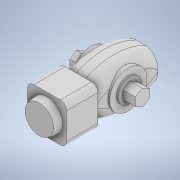
# Autodesk Inventor part: Weapon-Healing-Body
Saved by Autodesk Inventor 2020 (Build 240168000, 168)
## iProperties
Created: 2019-12-02
Part Number: Weapon-Healing-Body
Material: Generic
Document SubType Name: Modeling
Designer: vifly_01
Density: 1 g/cm^3
Appearance: Default
Author: vifly_01
Autodesk Inventor part; units mm, degrees
ref_plane "YZ Plane" through (0, 0, 0) normal (1, 0, 0) x (0, 1, 0)
ref_plane "XZ Plane" through (0, 0, 0) normal (0, 1, 0) x (-1, 0, 0)
ref_plane "XY Plane" through (0, 0, 0) normal (0, 0, 1) x (1, 0, 0)
sketch "Sketch1" plane through (0, 0, 0) normal (0, 0, 1) x (1, 0, 0)
  circle A0 centre (0, 0) radius 5
  dimension "d0" = 10
  constraints: 1 centre point, 1 coincident
  measures "d0" diameter of A0
extrude "Extrusion1" add sketch "Sketch1" along normal blind 2.5 draft -10
sketch "Sketch2" plane through (0, 0, 0) normal (0, 0, -1) x (-1, 0, 0)
  line L0 (-6.25, -6.25) -> (6.25, -6.25)
  line L1 (6.25, -6.25) -> (6.25, 6.25)
  line L2 (6.25, 6.25) -> (-6.25, 6.25)
  line L3 (-6.25, 6.25) -> (-6.25, -6.25)
  line L4 (-6.25, -6.25) -> (6.25, 6.25) construction
  line L5 (6.25, -6.25) -> (-6.25, 6.25) construction
  point P0 (0, 0)
  dimension "d3" = 12.5
  dimension "d4" = 12.5
  constraints: 12 end point, 2 midpoint, 2 parallel, 1 horizontal, 1 perpendicular
  measures "d3" distance of L2.end L1.end
  measures "d4" distance of L1.end L0.end
extrude "Extrusion2" add sketch "Sketch2" along normal blind 10
sketch "Sketch3" plane through (0, 0, 0) normal (1, 0, 0) x (0, 1, 0)
  line L0 (7.5, -10) -> (7.5, -30)
  line L1 (7.5, -30) -> (-7.5, -30)
  line L2 (-7.5, -30) -> (-7.5, -10)
  line L3 (-7.5, -10) -> (7.5, -10)
  point P0 (0, 0)
  dimension "d7" = 20
  dimension "d8" = 15
  constraints: 8 end point, 2 parallel, 1 perpendicular, 1 vertical
  measures "d7" distance of L0.start L0.end
  measures "d8" distance of L0.end L1.end
extrude "Extrusion3" add sketch "Sketch3" along normal mid plane 11
sketch "Sketch4" plane through (0, 0, 0) normal (1, 0, 0) x (0, 1, 0)
  line L0 (7.5, -30) -> (-7.5, -30) projected
  line L1 (-6.25, -10) -> (6.25, -10) projected
  line L2 (7.5, -30) -> (7.5, -10) projected
  line L3 (-6.25, -10) -> (6.25, -10) projected
  arc A0 (5, -30) -> (5, -10) centre (-13.75, -20) ccw
  line L4 (5, -10) -> (5, -30) construction
  line L5 (5, -10) -> (25, -10) construction
  arc A1 (-5, -10) -> (-5, -30) centre (13.75, -20) ccw
  line L6 (-5, -10) -> (-5, -30) construction
  line L7 (-5, -10) -> (15, -10) construction
  line L8 (6.25, -10) -> (7.5, -10) projected
  line L9 (5, -10) -> (7.5, -10)
  line L10 (7.5, -10) -> (7.5, -20)
  line L11 (7.5, -10) -> (7.5, -30) projected
  line L12 (7.5, -20) -> (7.5, -30)
  line L13 (7.5, -30) -> (5, -30)
  line L14 (-7.5, -30) -> (-7.5, -10) projected
  line L15 (-5, -30) -> (-7.5, -30)
  line L16 (-7.5, -30) -> (-7.5, -20)
  line L17 (-7.5, -10) -> (-6.25, -10) projected
  line L18 (-7.5, -20) -> (-7.5, -10)
  line L19 (-7.5, -10) -> (-5, -10)
  point P0 (0, 0)
  point P1 (-7.5, -20)
  point P2 (-5, -10)
  point P3 (5, -10)
  point P4 (7.5, -20)
  dimension "d11" = 90
  dimension "d12" = 90
  constraints: 24 end point, 5 point on circle, 4 point on line, 3 collinear, 3 horizontal, 2 centre point, 2 perpendicular, 2 vertical, 1 midpoint
  measures "d11" angle of L4 L5
  measures "d12" angle of L6 L7
extrude "Extrusion4" cut sketch "Sketch4" along normal mid plane 11 contours L0 A0 L2 | A0 L1 L8 L2 | L0 L14 A1 | L14 L17 L1 A1
fillet "Fillet1" radius 2 4 edges at (6.25, 6.25, -5) (6.25, -6.25, -5) (-6.25, 6.25, -5) (-6.25, -6.25, -5)
fillet "Fillet2" radius 4 4 edges at (5.5, 7.5, -20) (5.5, -7.5, -20) (-5.5, -7.5, -20) (-5.5, 7.5, -20)
sketch "Sketch5" plane through (5.5, 0, 0) normal (1, 0, 0) x (0, 0, -1)
  circle A0 centre (20, 0) radius 6
  point P0 (0, 0)
  dimension "d17" = 12
  constraints: 1 centre point
  measures "d17" diameter of A0
extrude "Extrusion5" add sketch "Sketch5" against normal blind 0.9
sketch "Sketch6" plane through (5.5, 0, 0) normal (1, 0, 0) x (0, 0, -1)
  circle A0 centre (20, 0) radius 6
  point P0 (0, 0)
  constraints: 1 centre point
extrude "Extrusion6" add sketch "Sketch6" along normal blind 0.5
sketch "Sketch9" plane through (6, 0, -20) normal (1, 0, 0) x (0, 0, -1)
  circle A0 centre (0, 0) radius 3.75
  point P0 (-20, 0)
  dimension "d26" = 7.5
  constraints: 1 centre point
  measures "d26" diameter of A0
extrude "Extrusion9" add sketch "Sketch9" along normal blind 0.5
sketch "Sketch10" plane through (6.5, 0, -20) normal (1, 0, 0) x (0, 0, -1)
  line L0 (0.0215, 2.6293) -> (2.2986, 1.3147)
  line L1 (2.2986, 1.3147) -> (2.2986, -1.3147)
  line L2 (2.2986, -1.3147) -> (0.0215, -2.6293)
  line L3 (0.0215, -2.6293) -> (-2.2556, -1.3147)
  line L4 (-2.2556, -1.3147) -> (-2.2556, 1.3147)
  line L5 (-2.2556, 1.3147) -> (0.0215, 2.6293)
  point P0 (-20, 0)
  point P1 (0.0215, 0)
  constraints: 12 end point, 1 vertical alignment, 13 other
extrude "Extrusion10" add sketch "Sketch10" along normal blind 4
mirror "Mirror1" about plane through (0, 0, 0) normal (1, 0, 0) of "Extrusion5", "Extrusion6", "Extrusion9", "Extrusion10"
equation "\"d4\" = d3"
body "Solid1"
